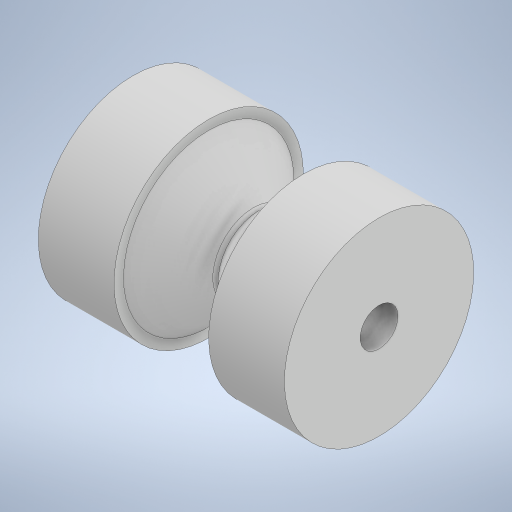
# Autodesk Inventor part: guideWheel
Saved by Autodesk Inventor 2024 (Build 280153000, 153)
## iProperties
Created: 2024-03-27
Part Number: guideWheel
Material: Generic
Document SubType Name: Modeling
Designer: Albin
Density: 1 g/cm^3
Appearance: Default
Author: Albin
Autodesk Inventor part; units mm, degrees
ref_plane "YZ Plane" through (0, 0, 0) normal (1, 0, 0) x (0, 1, 0)
ref_plane "XZ Plane" through (0, 0, 0) normal (0, 1, 0) x (-1, 0, 0)
ref_plane "XY Plane" through (0, 0, 0) normal (0, 0, 1) x (1, 0, 0)
sketch "Sketch2" plane through (0, 0, 0) normal (0, 0, 1) x (1, 0, 0)
  line L0 (0, 0) -> (-32.5, 0)
  line L1 (-32.5, 0) -> (-32.5, 25)
  line L2 (-32.5, 25) -> (-12.5, 25)
  line L3 (-12.5, 25) -> (-12.5, 22.5)
  line L4 (-12.5, 22.5) -> (12.5, 22.5)
  line L5 (12.5, 22.5) -> (12.5, 25)
  line L6 (12.5, 25) -> (32.5, 25)
  line L7 (32.5, 25) -> (32.5, 0)
  line L8 (32.5, 0) -> (0, 0)
  line L9 (-12.5, 22.5) -> (0, 10)
  line L10 (0, 10) -> (12.5, 22.5)
  line L11 (-45.5, 0) -> (45.5, 0) projected
  point P0 (0, 22.5)
  dimension "d1" = 20
  dimension "d2" = 65
  dimension "d4" = 25
  dimension "d5" = 45
  dimension "d6" = 45
  dimension "d7" = 5
  constraints: 22 end point, 7 perpendicular, 3 point on line, 2 collinear, 1 horizontal, 1 midpoint
  measures "d1" distance of L5.end L6.end
  measures "d2" distance between parallel lines of L1 L7
  measures "d4" distance of L6.end L7.end
  measures "d5" angle of L4 L10
  measures "d6" angle of L4 L9
  measures "d7" diameter of L6 L4
revolve "Revolution1" add sketch "Sketch2" angle 360 about axis through (-10, 0, 0) along (1, 0, 0) contours L0 L1 L2 L3 L9 L10 L5 L6 L7 L8
fillet "Fillet1" radius 1 1 edges at (0, -10, 0)
sketch "Sketch3" plane through (-32.5, 0, 0) normal (-1, 0, 0) x (0, 0, 1)
  circle A0 centre (0, 0) radius 5
  dimension "d10" = 10
  constraints: 1 centre point, 1 coincident
  measures "d10" diameter of A0
extrude "Extrusion1" cut sketch "Sketch3" against normal through all
sketch "Sketch5" plane through (0, 0, 0) normal (0, 1, 0) x (-1, 0, 0)
  line L0 (-32.5, 25) -> (-32.5, -25) projected
  line L1 (-32.5, 0) -> (32.6883, 0)
  line L2 (-12.5, 25) -> (-32.5, 25) projected
  line L3 (-22.5, 25) -> (-22.5, -25)
  line L4 (-12.5, -25) -> (-32.5, -25) projected
  line L5 (32.5, 25) -> (12.5, 25) projected
  line L6 (22.5, 25) -> (22.5, -25)
  line L7 (32.5, -25) -> (12.5, -25) projected
  circle A0 centre (-22.5, 0) radius 2.75
  point P0 (0, 0)
  dimension "d13" = 5.5
  constraints: 6 end point, 6 midpoint, 1 centre point, 1 horizontal
  measures "d13" diameter of A0
extrude "Extrusion2" cut sketch "Sketch5" against normal through all contours A0 L3 L1 | L1 L3 A0 | A0 L1 L3 | L1 A0 L3
body "Solid1"
